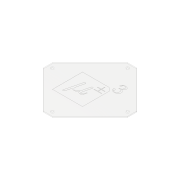
# Autodesk Inventor part: separatingPanels
Saved by Autodesk Inventor 2016 SP2 (Build 200236200, 236)
## iProperties
Created: 2016-07-21
Part Number: separatingPanels
Material: Polycarbonate, Clear
Document SubType Name: Modeling
Designer: Jonathan
Density: 1.2 g/cm^3
Appearance: Polycarbonate - Clear
Author: Jonathan
Autodesk Inventor part; units mm, degrees
(part 1 of 2)
ref_plane "YZ Plane" through (0, 0, 0) normal (1, 0, 0) x (0, 1, 0)
ref_plane "XZ Plane" through (0, 0, 0) normal (0, 1, 0) x (-1, 0, 0)
ref_plane "XY Plane" through (0, 0, 0) normal (0, 0, 1) x (1, 0, 0)
sketch "logo" plane through (0, 0, 0) normal (0, 0, 1) x (1, 0, 0)
  line L0 (123.8453, -88.283) -> (75.9446, -136.1837)
  line L1 (75.9446, -136.1837) -> (28.0439, -88.283)
  line L2 (28.0439, -88.283) -> (70.5564, -45.7705)
  spline S0 degree 3 poles (70.5564, -45.7705) (74.7474, -45.7705) (77.1417, -45.7705) (81.3327, -45.7705) knots 3 3 3 3 4 4 4 4
  line L3 (70.5564, -45.7705) -> (74.7474, -45.7705) construction
  line L4 (74.7474, -45.7705) -> (77.1417, -45.7705) construction
  line L5 (77.1417, -45.7705) -> (81.3327, -45.7705) construction
  line L6 (81.3327, -45.7705) -> (123.8453, -88.283)
  line L7 (135.6748, -1.3088) -> (16.9721, -1.3088)
  line L8 (16.9721, -1.3088) -> (1.3229, -16.958)
  line L9 (1.3229, -16.958) -> (1.3229, -135.6572)
  line L10 (1.3229, -135.6572) -> (16.9721, -151.3099)
  line L11 (16.9721, -151.3099) -> (135.6748, -151.3099)
  line L12 (135.6748, -151.3099) -> (151.324, -135.6572)
  line L13 (151.324, -135.6572) -> (151.324, -16.958)
  line L14 (151.324, -16.958) -> (135.6748, -1.3088)
  spline S1 degree 3 poles (16.2172, -139.1638) (14.7002, -139.1638) (13.4691, -137.9326) (13.4691, -136.4121) (13.4691, -134.8952) (14.7002, -133.664) (16.2172, -133.664) (17.7377, -133.664) (18.9689, -134.8952) (18.9689, -136.4121) (18.9689, -137.9326) (17.7377, -139.1638) (16.2172, -139.1638) knots 0 0 0 0 1 1 1 2 2 2 3 3 3 4 4 4 4
  line L15 (16.2172, -139.1638) -> (14.7002, -139.1638) construction
  line L16 (14.7002, -139.1638) -> (13.4691, -137.9326) construction
  line L17 (13.4691, -137.9326) -> (13.4691, -136.4121) construction
  line L18 (13.4691, -136.4121) -> (13.4691, -134.8952) construction
  line L19 (13.4691, -134.8952) -> (14.7002, -133.664) construction
  line L20 (14.7002, -133.664) -> (16.2172, -133.664) construction
  line L21 (16.2172, -133.664) -> (17.7377, -133.664) construction
  line L22 (17.7377, -133.664) -> (18.9689, -134.8952) construction
  line L23 (18.9689, -134.8952) -> (18.9689, -136.4121) construction
  line L24 (18.9689, -136.4121) -> (18.9689, -137.9326) construction
  line L25 (18.9689, -137.9326) -> (17.7377, -139.1638) construction
  line L26 (17.7377, -139.1638) -> (16.2172, -139.1638) construction
  spline S2 degree 3 poles (16.2172, -18.9547) (14.7002, -18.9547) (13.4691, -17.7236) (13.4691, -16.2031) (13.4691, -14.6861) (14.7002, -13.4549) (16.2172, -13.4549) (17.7377, -13.4549) (18.9689, -14.6861) (18.9689, -16.2031) (18.9689, -17.7236) (17.7377, -18.9547) (16.2172, -18.9547) knots 0 0 0 0 1 1 1 2 2 2 3 3 3 4 4 4 4
  line L27 (16.2172, -18.9547) -> (14.7002, -18.9547) construction
  line L28 (14.7002, -18.9547) -> (13.4691, -17.7236) construction
  line L29 (13.4691, -17.7236) -> (13.4691, -16.2031) construction
  line L30 (13.4691, -16.2031) -> (13.4691, -14.6861) construction
  line L31 (13.4691, -14.6861) -> (14.7002, -13.4549) construction
  line L32 (14.7002, -13.4549) -> (16.2172, -13.4549) construction
  line L33 (16.2172, -13.4549) -> (17.7377, -13.4549) construction
  line L34 (17.7377, -13.4549) -> (18.9689, -14.6861) construction
  line L35 (18.9689, -14.6861) -> (18.9689, -16.2031) construction
  line L36 (18.9689, -16.2031) -> (18.9689, -17.7236) construction
  line L37 (18.9689, -17.7236) -> (17.7377, -18.9547) construction
  line L38 (17.7377, -18.9547) -> (16.2172, -18.9547) construction
  spline S3 degree 3 poles (136.4262, -139.1638) (134.9093, -139.1638) (133.6781, -137.9326) (133.6781, -136.4121) (133.6781, -134.8952) (134.9093, -133.664) (136.4262, -133.664) (137.9467, -133.664) (139.1779, -134.8952) (139.1779, -136.4121) (139.1779, -137.9326) (137.9467, -139.1638) (136.4262, -139.1638) knots 0 0 0 0 1 1 1 2 2 2 3 3 3 4 4 4 4
  line L39 (136.4262, -139.1638) -> (134.9093, -139.1638) construction
  line L40 (134.9093, -139.1638) -> (133.6781, -137.9326) construction
  line L41 (133.6781, -137.9326) -> (133.6781, -136.4121) construction
  line L42 (133.6781, -136.4121) -> (133.6781, -134.8952) construction
  line L43 (133.6781, -134.8952) -> (134.9093, -133.664) construction
  line L44 (134.9093, -133.664) -> (136.4262, -133.664) construction
  line L45 (136.4262, -133.664) -> (137.9467, -133.664) construction
  line L46 (137.9467, -133.664) -> (139.1779, -134.8952) construction
  line L47 (139.1779, -134.8952) -> (139.1779, -136.4121) construction
  line L48 (139.1779, -136.4121) -> (139.1779, -137.9326) construction
  line L49 (139.1779, -137.9326) -> (137.9467, -139.1638) construction
  line L50 (137.9467, -139.1638) -> (136.4262, -139.1638) construction
  spline S4 degree 3 poles (136.4262, -18.9547) (134.9093, -18.9547) (133.6781, -17.7236) (133.6781, -16.2031) (133.6781, -14.6861) (134.9093, -13.4549) (136.4262, -13.4549) (137.9467, -13.4549) (139.1779, -14.6861) (139.1779, -16.2031) (139.1779, -17.7236) (137.9467, -18.9547) (136.4262, -18.9547) knots 0 0 0 0 1 1 1 2 2 2 3 3 3 4 4 4 4
  line L51 (136.4262, -18.9547) -> (134.9093, -18.9547) construction
  line L52 (134.9093, -18.9547) -> (133.6781, -17.7236) construction
  line L53 (133.6781, -17.7236) -> (133.6781, -16.2031) construction
  line L54 (133.6781, -16.2031) -> (133.6781, -14.6861) construction
  line L55 (133.6781, -14.6861) -> (134.9093, -13.4549) construction
  line L56 (134.9093, -13.4549) -> (136.4262, -13.4549) construction
  line L57 (136.4262, -13.4549) -> (137.9467, -13.4549) construction
  line L58 (137.9467, -13.4549) -> (139.1779, -14.6861) construction
  line L59 (139.1779, -14.6861) -> (139.1779, -16.2031) construction
  line L60 (139.1779, -16.2031) -> (139.1779, -17.7236) construction
  line L61 (139.1779, -17.7236) -> (137.9467, -18.9547) construction
  line L62 (137.9467, -18.9547) -> (136.4262, -18.9547) construction
  spline S5 degree 3 poles (62.3098, -86.8642) (61.6869, -85.6876) (60.3719, -83.542) (60.1643, -83.3344) knots 0 0 0 0 1 1 1 1
  line L63 (62.3098, -86.8642) -> (61.6869, -85.6876) construction
  line L64 (61.6869, -85.6876) -> (60.3719, -83.542) construction
  line L65 (60.3719, -83.542) -> (60.1643, -83.3344) construction
  spline S6 degree 3 poles (60.1643, -83.3344) (59.4029, -82.573) (58.434, -82.7115) (57.6726, -83.4728) knots 1 1 1 1 2 2 2 2
  line L66 (60.1643, -83.3344) -> (59.4029, -82.573) construction
  line L67 (59.4029, -82.573) -> (58.434, -82.7115) construction
  line L68 (58.434, -82.7115) -> (57.6726, -83.4728) construction
  spline S7 degree 3 poles (57.6726, -83.4728) (57.6034, -83.542) (56.4268, -84.857) (57.5342, -86.795) knots 2 2 2 2 3 3 3 3
  line L69 (57.6726, -83.4728) -> (57.6034, -83.542) construction
  line L70 (57.6034, -83.542) -> (56.4268, -84.857) construction
  line L71 (56.4268, -84.857) -> (57.5342, -86.795) construction
  line L72 (57.5342, -86.795) -> (76.7059, -118.7017)
  spline S8 degree 3 poles (76.7059, -118.7017) (77.1212, -119.3938) (77.1904, -119.463) (77.3288, -119.6015) knots 4 4 4 4 5 5 5 5
  line L73 (76.7059, -118.7017) -> (77.1212, -119.3938) construction
  line L74 (77.1212, -119.3938) -> (77.1904, -119.463) construction
  line L75 (77.1904, -119.463) -> (77.3288, -119.6015) construction
  spline S9 degree 3 poles (77.3288, -119.6015) (77.9517, -120.2244) (78.9899, -120.2936) (79.7513, -119.5322) (80.651, -118.6325) (80.3742, -117.2482) (80.3049, -117.0406) knots 5 5 5 5 6 6 6 7 7 7 7
  line L76 (77.3288, -119.6015) -> (77.9517, -120.2244) construction
  line L77 (77.9517, -120.2244) -> (78.9899, -120.2936) construction
  line L78 (78.9899, -120.2936) -> (79.7513, -119.5322) construction
  line L79 (79.7513, -119.5322) -> (80.651, -118.6325) construction
  line L80 (80.651, -118.6325) -> (80.3742, -117.2482) construction
  line L81 (80.3742, -117.2482) -> (80.3049, -117.0406) construction
  spline S10 degree 3 poles (80.3049, -117.0406) (80.1665, -116.4869) (78.367, -113.58) (73.2453, -105.1361) knots 7 7 7 7 8 8 8 8
  line L82 (80.3049, -117.0406) -> (80.1665, -116.4869) construction
  line L83 (80.1665, -116.4869) -> (78.367, -113.58) construction
  line L84 (78.367, -113.58) -> (73.2453, -105.1361) construction
  spline S11 degree 3 poles (73.2453, -105.1361) (75.8754, -104.8593) (78.0902, -103.0598) (78.9207, -102.2292) (82.0352, -99.1147) (81.7584, -95.3773) (81.5508, -93.0933) knots 8 8 8 8 9 9 9 10 10 10 10
  line L85 (73.2453, -105.1361) -> (75.8754, -104.8593) construction
  line L86 (75.8754, -104.8593) -> (78.0902, -103.0598) construction
  line L87 (78.0902, -103.0598) -> (78.9207, -102.2292) construction
  line L88 (78.9207, -102.2292) -> (82.0352, -99.1147) construction
  line L89 (82.0352, -99.1147) -> (81.7584, -95.3773) construction
  line L90 (81.7584, -95.3773) -> (81.5508, -93.0933) construction
  spline S12 degree 3 poles (81.5508, -93.0933) (83.9732, -94.6851) (86.8801, -94.2699) (88.818, -92.3319) (90.3407, -90.8093) (90.3407, -88.7329) (89.6486, -86.6565) knots 10 10 10 10 11 11 11 12 12 12 12
  line L91 (81.5508, -93.0933) -> (83.9732, -94.6851) construction
  line L92 (83.9732, -94.6851) -> (86.8801, -94.2699) construction
  line L93 (86.8801, -94.2699) -> (88.818, -92.3319) construction
  line L94 (88.818, -92.3319) -> (90.3407, -90.8093) construction
  line L95 (90.3407, -90.8093) -> (90.3407, -88.7329) construction
  line L96 (90.3407, -88.7329) -> (89.6486, -86.6565) construction
  spline S13 degree 3 poles (89.6486, -86.6565) (88.818, -84.3033) (86.6725, -81.0504) (86.6032, -80.9812) knots 12 12 12 12 13 13 13 13
  line L97 (89.6486, -86.6565) -> (88.818, -84.3033) construction
  line L98 (88.818, -84.3033) -> (86.6725, -81.0504) construction
  line L99 (86.6725, -81.0504) -> (86.6032, -80.9812) construction
  spline S14 degree 3 poles (86.6032, -80.9812) (86.1188, -80.4967) (85.7035, -80.9119) (85.5651, -81.0504) (85.1498, -81.4656) (85.2882, -81.7425) (85.7727, -82.5038) knots 13 13 13 13 14 14 14 15 15 15 15
  line L100 (86.6032, -80.9812) -> (86.1188, -80.4967) construction
  line L101 (86.1188, -80.4967) -> (85.7035, -80.9119) construction
  line L102 (85.7035, -80.9119) -> (85.5651, -81.0504) construction
  line L103 (85.5651, -81.0504) -> (85.1498, -81.4656) construction
  line L104 (85.1498, -81.4656) -> (85.2882, -81.7425) construction
  line L105 (85.2882, -81.7425) -> (85.7727, -82.5038) construction
  spline S15 degree 3 poles (85.7727, -82.5038) (87.9183, -86.0336) (89.7178, -89.4942) (87.9183, -91.2937) (86.7417, -92.4703) (85.4266, -91.4322) (84.5961, -90.6016) (83.6271, -89.6327) (82.0352, -87.0718) (80.7894, -85.1339) knots 15 15 15 15 16 16 16 17 17 17 18 18 18 18
  line L106 (85.7727, -82.5038) -> (87.9183, -86.0336) construction
  line L107 (87.9183, -86.0336) -> (89.7178, -89.4942) construction
  line L108 (89.7178, -89.4942) -> (87.9183, -91.2937) construction
  line L109 (87.9183, -91.2937) -> (86.7417, -92.4703) construction
  line L110 (86.7417, -92.4703) -> (85.4266, -91.4322) construction
  line L111 (85.4266, -91.4322) -> (84.5961, -90.6016) construction
  line L112 (84.5961, -90.6016) -> (83.6271, -89.6327) construction
  line L113 (83.6271, -89.6327) -> (82.0352, -87.0718) construction
  line L114 (82.0352, -87.0718) -> (80.7894, -85.1339) construction
  line L115 (80.7894, -85.1339) -> (77.2596, -79.1124)
  spline S16 degree 3 poles (77.2596, -79.1124) (76.7751, -78.3511) (75.5985, -76.2055) (75.0448, -75.375) (74.2143, -74.1292) (73.0377, -71.9836) (72.7608, -71.7068) knots 19 19 19 19 20 20 20 21 21 21 21
  line L116 (77.2596, -79.1124) -> (76.7751, -78.3511) construction
  line L117 (76.7751, -78.3511) -> (75.5985, -76.2055) construction
  line L118 (75.5985, -76.2055) -> (75.0448, -75.375) construction
  line L119 (75.0448, -75.375) -> (74.2143, -74.1292) construction
  line L120 (74.2143, -74.1292) -> (73.0377, -71.9836) construction
  line L121 (73.0377, -71.9836) -> (72.7608, -71.7068) construction
  spline S17 degree 3 poles (72.7608, -71.7068) (71.9995, -70.9454) (70.9613, -71.1531) (70.2692, -71.8452) (70.0616, -72.0528) (68.9542, -73.2986) (70.0616, -75.0981) knots 21 21 21 21 22 22 22 23 23 23 23
  line L122 (72.7608, -71.7068) -> (71.9995, -70.9454) construction
  line L123 (71.9995, -70.9454) -> (70.9613, -71.1531) construction
  line L124 (70.9613, -71.1531) -> (70.2692, -71.8452) construction
  line L125 (70.2692, -71.8452) -> (70.0616, -72.0528) construction
  line L126 (70.0616, -72.0528) -> (68.9542, -73.2986) construction
  line L127 (68.9542, -73.2986) -> (70.0616, -75.0981) construction
  line L128 (70.0616, -75.0981) -> (76.2907, -85.4799)
  spline S18 degree 3 poles (76.2907, -85.4799) (78.021, -88.1792) (79.336, -90.4632) (79.682, -91.0861) knots 24 24 24 24 25 25 25 25
  line L129 (76.2907, -85.4799) -> (78.021, -88.1792) construction
  line L130 (78.021, -88.1792) -> (79.336, -90.4632) construction
  line L131 (79.336, -90.4632) -> (79.682, -91.0861) construction
  spline S19 degree 3 poles (79.682, -91.0861) (79.8205, -91.363) (81.7584, -97.4536) (78.1594, -101.0526) (75.9446, -103.2674) (73.453, -102.8521) (71.0305, -100.4297) (69.7847, -99.1839) (68.8158, -97.6612) (67.916, -96.0694) knots 25 25 25 25 26 26 26 27 27 27 28 28 28 28
  line L132 (79.682, -91.0861) -> (79.8205, -91.363) construction
  line L133 (79.8205, -91.363) -> (81.7584, -97.4536) construction
  line L134 (81.7584, -97.4536) -> (78.1594, -101.0526) construction
  line L135 (78.1594, -101.0526) -> (75.9446, -103.2674) construction
  line L136 (75.9446, -103.2674) -> (73.453, -102.8521) construction
  line L137 (73.453, -102.8521) -> (71.0305, -100.4297) construction
  line L138 (71.0305, -100.4297) -> (69.7847, -99.1839) construction
  line L139 (69.7847, -99.1839) -> (68.8158, -97.6612) construction
  line L140 (68.8158, -97.6612) -> (67.916, -96.0694) construction
  line L141 (67.916, -96.0694) -> (62.3098, -86.8642)
  line L142 (76.7453, -58.3124) -> (81.6949, -53.3628)
  spline S20 degree 3 poles (81.6949, -53.3628) (81.9496, -53.1081) (82.3136, -52.7441) (81.9132, -52.3438) knots 1 1 1 1 2 2 2 2
  line L143 (81.6949, -53.3628) -> (81.9496, -53.1081) construction
  line L144 (81.9496, -53.1081) -> (82.3136, -52.7441) construction
  line L145 (82.3136, -52.7441) -> (81.9132, -52.3438) construction
  spline S21 degree 3 poles (81.9132, -52.3438) (81.5129, -51.9435) (81.149, -52.3074) (80.8942, -52.5622) knots 2 2 2 2 3 3 3 3
  line L146 (81.9132, -52.3438) -> (81.5129, -51.9435) construction
  line L147 (81.5129, -51.9435) -> (81.149, -52.3074) construction
  line L148 (81.149, -52.3074) -> (80.8942, -52.5622) construction
  line L149 (80.8942, -52.5622) -> (75.9446, -57.5118)
  line L150 (75.9446, -57.5118) -> (71.0678, -52.635)
  spline S22 degree 3 poles (71.0678, -52.635) (70.7766, -52.3438) (70.3763, -51.9435) (69.976, -52.3438) (69.5756, -52.7441) (69.9396, -53.1081) (70.1943, -53.3628) knots 5 5 5 5 6 6 6 7 7 7 7
  line L151 (71.0678, -52.635) -> (70.7766, -52.3438) construction
  line L152 (70.7766, -52.3438) -> (70.3763, -51.9435) construction
  line L153 (70.3763, -51.9435) -> (69.976, -52.3438) construction
  line L154 (69.976, -52.3438) -> (69.5756, -52.7441) construction
  line L155 (69.5756, -52.7441) -> (69.9396, -53.1081) construction
  line L156 (69.9396, -53.1081) -> (70.1943, -53.3628) construction
  line L157 (70.1943, -53.3628) -> (75.1439, -58.3124)
  line L158 (75.1439, -58.3124) -> (70.1943, -63.262)
  spline S23 degree 3 poles (70.1943, -63.262) (69.9396, -63.5168) (69.5392, -63.9171) (69.9396, -64.3175) knots 9 9 9 9 10 10 10 10
  line L159 (70.1943, -63.262) -> (69.9396, -63.5168) construction
  line L160 (69.9396, -63.5168) -> (69.5392, -63.9171) construction
  line L161 (69.5392, -63.9171) -> (69.9396, -64.3175) construction
  spline S24 degree 3 poles (69.9396, -64.3175) (70.3399, -64.7178) (70.7402, -64.3175) (70.995, -64.0627) knots 10 10 10 10 11 11 11 11
  line L162 (69.9396, -64.3175) -> (70.3399, -64.7178) construction
  line L163 (70.3399, -64.7178) -> (70.7402, -64.3175) construction
  line L164 (70.7402, -64.3175) -> (70.995, -64.0627) construction
  line L165 (70.995, -64.0627) -> (75.9446, -59.1131)
  line L166 (75.9446, -59.1131) -> (80.7486, -63.9171)
  line L167 (80.7486, -63.9171) -> (75.799, -68.8667)
  spline S25 degree 3 poles (75.799, -68.8667) (75.5443, -69.1215) (75.1439, -69.5218) (75.5443, -69.9222) knots 14 14 14 14 15 15 15 15
  line L168 (75.799, -68.8667) -> (75.5443, -69.1215) construction
  line L169 (75.5443, -69.1215) -> (75.1439, -69.5218) construction
  line L170 (75.1439, -69.5218) -> (75.5443, -69.9222) construction
  spline S26 degree 3 poles (75.5443, -69.9222) (75.9446, -70.3225) (76.3449, -69.9222) (76.5997, -69.6674) knots 15 15 15 15 16 16 16 16
  line L171 (75.5443, -69.9222) -> (75.9446, -70.3225) construction
  line L172 (75.9446, -70.3225) -> (76.3449, -69.9222) construction
  line L173 (76.3449, -69.9222) -> (76.5997, -69.6674) construction
  line L174 (76.5997, -69.6674) -> (87.2996, -58.9675)
  spline S27 degree 3 poles (87.2996, -58.9675) (87.5543, -58.7128) (87.9183, -58.3488) (87.5179, -57.9485) knots 17 17 17 17 18 18 18 18
  line L175 (87.2996, -58.9675) -> (87.5543, -58.7128) construction
  line L176 (87.5543, -58.7128) -> (87.9183, -58.3488) construction
  line L177 (87.9183, -58.3488) -> (87.5179, -57.9485) construction
  spline S28 degree 3 poles (87.5179, -57.9485) (87.1176, -57.5482) (86.7537, -57.9121) (86.4989, -58.1669) knots 18 18 18 18 19 19 19 19
  line L178 (87.5179, -57.9485) -> (87.1176, -57.5482) construction
  line L179 (87.1176, -57.5482) -> (86.7537, -57.9121) construction
  line L180 (86.7537, -57.9121) -> (86.4989, -58.1669) construction
  line L181 (86.4989, -58.1669) -> (81.5493, -63.1165)
  line L182 (81.5493, -63.1165) -> (76.7453, -58.3124)
  spline S29 degree 3 poles (75.3605, -28.3562) (77.4048, -26.312) (80.2668, -26.2535) (83.0704, -29.0571) (86.2828, -32.2696) (85.3483, -35.19) (83.8881, -36.6502) (82.8368, -37.7015) (80.2084, -39.7458) (77.58, -39.2202) knots 0 0 0 0 1 1 1 2 2 2 3 3 3 3
  line L183 (75.3605, -28.3562) -> (77.4048, -26.312) construction
  line L184 (77.4048, -26.312) -> (80.2668, -26.2535) construction
  line L185 (80.2668, -26.2535) -> (83.0704, -29.0571) construction
  line L186 (83.0704, -29.0571) -> (86.2828, -32.2696) construction
  line L187 (86.2828, -32.2696) -> (85.3483, -35.19) construction
  line L188 (85.3483, -35.19) -> (83.8881, -36.6502) construction
  line L189 (83.8881, -36.6502) -> (82.8368, -37.7015) construction
  line L190 (82.8368, -37.7015) -> (80.2084, -39.7458) construction
  line L191 (80.2084, -39.7458) -> (77.58, -39.2202) construction
  spline S30 degree 3 poles (77.58, -39.2202) (78.8066, -37.9936) (78.2225, -36.8254) (77.6384, -36.2413) (76.8207, -35.4236) (75.5941, -35.482) (74.7764, -36.2998) (74.0755, -37.0007) (73.7835, -38.2272) (74.8348, -39.2786) (77.288, -41.7317) (81.5518, -40.622) (84.7058, -37.4679) (88.3271, -33.8466) (88.3855, -28.8819) (85.8156, -26.312) (83.7713, -24.2677) (80.0916, -23.8588) (76.6455, -26.1367) knots 3 3 3 3 4 4 4 5 5 5 6 6 6 7 7 7 8 8 8 9 9 9 9
  line L192 (77.58, -39.2202) -> (78.8066, -37.9936) construction
  line L193 (78.8066, -37.9936) -> (78.2225, -36.8254) construction
  line L194 (78.2225, -36.8254) -> (77.6384, -36.2413) construction
  line L195 (77.6384, -36.2413) -> (76.8207, -35.4236) construction
  line L196 (76.8207, -35.4236) -> (75.5941, -35.482) construction
  line L197 (75.5941, -35.482) -> (74.7764, -36.2998) construction
  line L198 (74.7764, -36.2998) -> (74.0755, -37.0007) construction
  line L199 (74.0755, -37.0007) -> (73.7835, -38.2272) construction
  line L200 (73.7835, -38.2272) -> (74.8348, -39.2786) construction
  line L201 (74.8348, -39.2786) -> (77.288, -41.7317) construction
  line L202 (77.288, -41.7317) -> (81.5518, -40.622) construction
  line L203 (81.5518, -40.622) -> (84.7058, -37.4679) construction
  line L204 (84.7058, -37.4679) -> (88.3271, -33.8466) construction
  line L205 (88.3271, -33.8466) -> (88.3855, -28.8819) construction
  line L206 (88.3855, -28.8819) -> (85.8156, -26.312) construction
  line L207 (85.8156, -26.312) -> (83.7713, -24.2677) construction
  line L208 (83.7713, -24.2677) -> (80.0916, -23.8588) construction
  line L209 (80.0916, -23.8588) -> (76.6455, -26.1367) construction
  spline S31 degree 3 poles (76.6455, -26.1367) (78.3393, -22.457) (77.4048, -19.5366) (75.7694, -17.9012) (73.7251, -15.8569) (69.8701, -16.6746) (66.9497, -19.595) (64.0877, -22.457) (63.27, -26.0783) (65.3727, -28.181) (66.2488, -29.0571) (67.3002, -28.9403) (68.0595, -28.181) (68.8772, -27.3633) (68.8188, -26.2535) (68.1179, -25.5526) (67.3586, -24.7933) (66.2488, -24.7349) (65.3727, -25.4942) knots 9 9 9 9 10 10 10 11 11 11 12 12 12 13 13 13 14 14 14 15 15 15 15
  line L210 (76.6455, -26.1367) -> (78.3393, -22.457) construction
  line L211 (78.3393, -22.457) -> (77.4048, -19.5366) construction
  line L212 (77.4048, -19.5366) -> (75.7694, -17.9012) construction
  line L213 (75.7694, -17.9012) -> (73.7251, -15.8569) construction
  line L214 (73.7251, -15.8569) -> (69.8701, -16.6746) construction
  line L215 (69.8701, -16.6746) -> (66.9497, -19.595) construction
  line L216 (66.9497, -19.595) -> (64.0877, -22.457) construction
  line L217 (64.0877, -22.457) -> (63.27, -26.0783) construction
  line L218 (63.27, -26.0783) -> (65.3727, -28.181) construction
  line L219 (65.3727, -28.181) -> (66.2488, -29.0571) construction
  line L220 (66.2488, -29.0571) -> (67.3002, -28.9403) construction
  line L221 (67.3002, -28.9403) -> (68.0595, -28.181) construction
  line L222 (68.0595, -28.181) -> (68.8772, -27.3633) construction
  line L223 (68.8772, -27.3633) -> (68.8188, -26.2535) construction
  line L224 (68.8188, -26.2535) -> (68.1179, -25.5526) construction
  line L225 (68.1179, -25.5526) -> (67.3586, -24.7933) construction
  line L226 (67.3586, -24.7933) -> (66.2488, -24.7349) construction
  line L227 (66.2488, -24.7349) -> (65.3727, -25.4942) construction
  spline S32 degree 3 poles (65.3727, -25.4942) (65.1975, -23.45) (66.6577, -21.4057) (67.6506, -20.4127) (68.8188, -19.2446) (71.0383, -18.1932) (73.2578, -20.4127) (74.3676, -21.5225) (75.2437, -23.0995) (75.3021, -24.5597) knots 15 15 15 15 16 16 16 17 17 17 18 18 18 18
  line L228 (65.3727, -25.4942) -> (65.1975, -23.45) construction
  line L229 (65.1975, -23.45) -> (66.6577, -21.4057) construction
  line L230 (66.6577, -21.4057) -> (67.6506, -20.4127) construction
  line L231 (67.6506, -20.4127) -> (68.8188, -19.2446) construction
  line L232 (68.8188, -19.2446) -> (71.0383, -18.1932) construction
  line L233 (71.0383, -18.1932) -> (73.2578, -20.4127) construction
  line L234 (73.2578, -20.4127) -> (74.3676, -21.5225) construction
  line L235 (74.3676, -21.5225) -> (75.2437, -23.0995) construction
  line L236 (75.2437, -23.0995) -> (75.3021, -24.5597) construction
  spline S33 degree 3 poles (75.3021, -24.5597) (75.4773, -26.3704) (74.7764, -27.1881) (73.6083, -28.5899) (73.0242, -29.2908) (72.9658, -29.3492) (72.849, -29.466) (72.7906, -29.5244) (72.6153, -29.8164) (72.9074, -30.1085) knots 18 18 18 18 19 19 19 20 20 20 21 21 21 21
  line L237 (75.3021, -24.5597) -> (75.4773, -26.3704) construction
  line L238 (75.4773, -26.3704) -> (74.7764, -27.1881) construction
  line L239 (74.7764, -27.1881) -> (73.6083, -28.5899) construction
  line L240 (73.6083, -28.5899) -> (73.0242, -29.2908) construction
  line L241 (73.0242, -29.2908) -> (72.9658, -29.3492) construction
  line L242 (72.9658, -29.3492) -> (72.849, -29.466) construction
  line L243 (72.849, -29.466) -> (72.7906, -29.5244) construction
  line L244 (72.7906, -29.5244) -> (72.6153, -29.8164) construction
  line L245 (72.6153, -29.8164) -> (72.9074, -30.1085) construction
  spline S34 degree 3 poles (72.9074, -30.1085) (73.2578, -30.4589) (73.4914, -30.2253) (73.9587, -29.758) knots 21 21 21 21 22 22 22 22
  line L246 (72.9074, -30.1085) -> (73.2578, -30.4589) construction
  line L247 (73.2578, -30.4589) -> (73.4914, -30.2253) construction
  line L248 (73.4914, -30.2253) -> (73.9587, -29.758) construction
  line L249 (73.9587, -29.758) -> (75.3605, -28.3562)
  point P0 (76.1833, -66.2121)
sketch "mu" plane through (0, 0, 0) normal (0, 0, 1) x (1, 0, 0)
  spline S0 degree 3 poles (-17.3729, 2.4446) (-16.9814, 3.7171) (-16.3941, 6.1641) (-16.3941, 6.4577) knots 0 0 0 0 1 1 1 1
  line L0 (-17.3729, 2.4446) -> (-16.9814, 3.7171) construction
  line L1 (-16.9814, 3.7171) -> (-16.3941, 6.1641) construction
  line L2 (-16.3941, 6.1641) -> (-16.3941, 6.4577) construction
  spline S1 degree 3 poles (-16.3941, 6.4577) (-16.3941, 7.5344) (-17.1772, 8.1217) (-18.2539, 8.1217) knots 1 1 1 1 2 2 2 2
  line L3 (-16.3941, 6.4577) -> (-16.3941, 7.5344) construction
  line L4 (-16.3941, 7.5344) -> (-17.1772, 8.1217) construction
  line L5 (-17.1772, 8.1217) -> (-18.2539, 8.1217) construction
  spline S2 degree 3 poles (-18.2539, 8.1217) (-18.3517, 8.1217) (-20.1136, 8.0238) (-20.7009, 5.8705) knots 2 2 2 2 3 3 3 3
  line L6 (-18.2539, 8.1217) -> (-18.3517, 8.1217) construction
  line L7 (-18.3517, 8.1217) -> (-20.1136, 8.0238) construction
  line L8 (-20.1136, 8.0238) -> (-20.7009, 5.8705) construction
  line L9 (-20.7009, 5.8705) -> (-29.7059, -30.2475)
  spline S3 degree 3 poles (-29.7059, -30.2475) (-29.9017, -31.0305) (-29.9017, -31.1284) (-29.9017, -31.3241) knots 4 4 4 4 5 5 5 5
  line L10 (-29.7059, -30.2475) -> (-29.9017, -31.0305) construction
  line L11 (-29.9017, -31.0305) -> (-29.9017, -31.1284) construction
  line L12 (-29.9017, -31.1284) -> (-29.9017, -31.3241) construction
  spline S4 degree 3 poles (-29.9017, -31.3241) (-29.9017, -32.2051) (-29.2165, -32.9881) (-28.1398, -32.9881) (-26.8674, -32.9881) (-26.0843, -31.8136) (-25.9864, -31.6178) knots 5 5 5 5 6 6 6 7 7 7 7
  line L13 (-29.9017, -31.3241) -> (-29.9017, -32.2051) construction
  line L14 (-29.9017, -32.2051) -> (-29.2165, -32.9881) construction
  line L15 (-29.2165, -32.9881) -> (-28.1398, -32.9881) construction
  line L16 (-28.1398, -32.9881) -> (-26.8674, -32.9881) construction
  line L17 (-26.8674, -32.9881) -> (-26.0843, -31.8136) construction
  line L18 (-26.0843, -31.8136) -> (-25.9864, -31.6178) construction
  spline S5 degree 3 poles (-25.9864, -31.6178) (-25.6928, -31.1284) (-24.9098, -27.8004) (-22.5606, -18.2082) knots 7 7 7 7 8 8 8 8
  line L19 (-25.9864, -31.6178) -> (-25.6928, -31.1284) construction
  line L20 (-25.6928, -31.1284) -> (-24.9098, -27.8004) construction
  line L21 (-24.9098, -27.8004) -> (-22.5606, -18.2082) construction
  spline S6 degree 3 poles (-22.5606, -18.2082) (-20.5051, -19.8721) (-17.6666, -20.1658) (-16.492, -20.1658) (-12.0874, -20.1658) (-9.6404, -17.3272) (-8.1722, -15.5654) knots 8 8 8 8 9 9 9 10 10 10 10
  line L22 (-22.5606, -18.2082) -> (-20.5051, -19.8721) construction
  line L23 (-20.5051, -19.8721) -> (-17.6666, -20.1658) construction
  line L24 (-17.6666, -20.1658) -> (-16.492, -20.1658) construction
  line L25 (-16.492, -20.1658) -> (-12.0874, -20.1658) construction
  line L26 (-12.0874, -20.1658) -> (-9.6404, -17.3272) construction
  line L27 (-9.6404, -17.3272) -> (-8.1722, -15.5654) construction
  spline S7 degree 3 poles (-8.1722, -15.5654) (-7.5849, -18.4039) (-5.2358, -20.1658) (-2.4951, -20.1658) (-0.3417, -20.1658) (1.1265, -18.6976) (2.1053, -16.74) knots 10 10 10 10 11 11 11 12 12 12 12
  line L28 (-8.1722, -15.5654) -> (-7.5849, -18.4039) construction
  line L29 (-7.5849, -18.4039) -> (-5.2358, -20.1658) construction
  line L30 (-5.2358, -20.1658) -> (-2.4951, -20.1658) construction
  line L31 (-2.4951, -20.1658) -> (-0.3417, -20.1658) construction
  line L32 (-0.3417, -20.1658) -> (1.1265, -18.6976) construction
  line L33 (1.1265, -18.6976) -> (2.1053, -16.74) construction
  spline S8 degree 3 poles (2.1053, -16.74) (3.182, -14.4887) (3.965, -10.6714) (3.965, -10.5735) knots 12 12 12 12 13 13 13 13
  line L34 (2.1053, -16.74) -> (3.182, -14.4887) construction
  line L35 (3.182, -14.4887) -> (3.965, -10.6714) construction
  line L36 (3.965, -10.6714) -> (3.965, -10.5735) construction
  spline S9 degree 3 poles (3.965, -10.5735) (3.965, -9.8883) (3.3777, -9.8883) (3.182, -9.8883) (2.5947, -9.8883) (2.4968, -10.182) (2.301, -11.0629) knots 13 13 13 13 14 14 14 15 15 15 15
  line L37 (3.965, -10.5735) -> (3.965, -9.8883) construction
  line L38 (3.965, -9.8883) -> (3.3777, -9.8883) construction
  line L39 (3.3777, -9.8883) -> (3.182, -9.8883) construction
  line L40 (3.182, -9.8883) -> (2.5947, -9.8883) construction
  line L41 (2.5947, -9.8883) -> (2.4968, -10.182) construction
  line L42 (2.4968, -10.182) -> (2.301, -11.0629) construction
  spline S10 degree 3 poles (2.301, -11.0629) (1.3222, -15.076) (0.1477, -18.7955) (-2.3972, -18.7955) (-4.0612, -18.7955) (-4.257, -17.1315) (-4.257, -15.9569) (-4.257, -14.5866) (-3.5718, -11.6502) (-3.0824, -9.3989) knots 15 15 15 15 16 16 16 17 17 17 18 18 18 18
  line L43 (2.301, -11.0629) -> (1.3222, -15.076) construction
  line L44 (1.3222, -15.076) -> (0.1477, -18.7955) construction
  line L45 (0.1477, -18.7955) -> (-2.3972, -18.7955) construction
  line L46 (-2.3972, -18.7955) -> (-4.0612, -18.7955) construction
  line L47 (-4.0612, -18.7955) -> (-4.257, -17.1315) construction
  line L48 (-4.257, -17.1315) -> (-4.257, -15.9569) construction
  line L49 (-4.257, -15.9569) -> (-4.257, -14.5866) construction
  line L50 (-4.257, -14.5866) -> (-3.5718, -11.6502) construction
  line L51 (-3.5718, -11.6502) -> (-3.0824, -9.3989) construction
  line L52 (-3.0824, -9.3989) -> (-1.3205, -2.6452)
  spline S11 degree 3 poles (-1.3205, -2.6452) (-1.1248, -1.7642) (-0.4396, 0.5849) (-0.2438, 1.5637) (0.0498, 3.0319) (0.735, 5.381) (0.735, 5.7726) knots 19 19 19 19 20 20 20 21 21 21 21
  line L53 (-1.3205, -2.6452) -> (-1.1248, -1.7642) construction
  line L54 (-1.1248, -1.7642) -> (-0.4396, 0.5849) construction
  line L55 (-0.4396, 0.5849) -> (-0.2438, 1.5637) construction
  line L56 (-0.2438, 1.5637) -> (0.0498, 3.0319) construction
  line L57 (0.0498, 3.0319) -> (0.735, 5.381) construction
  line L58 (0.735, 5.381) -> (0.735, 5.7726) construction
  spline S12 degree 3 poles (0.735, 5.7726) (0.735, 6.8492) (-0.146, 7.4365) (-1.1248, 7.4365) (-1.4184, 7.4365) (-3.0824, 7.3386) (-3.5718, 5.2832) knots 21 21 21 21 22 22 22 23 23 23 23
  line L59 (0.735, 5.7726) -> (0.735, 6.8492) construction
  line L60 (0.735, 6.8492) -> (-0.146, 7.4365) construction
  line L61 (-0.146, 7.4365) -> (-1.1248, 7.4365) construction
  line L62 (-1.1248, 7.4365) -> (-1.4184, 7.4365) construction
  line L63 (-1.4184, 7.4365) -> (-3.0824, 7.3386) construction
  line L64 (-3.0824, 7.3386) -> (-3.5718, 5.2832) construction
  line L65 (-3.5718, 5.2832) -> (-6.5082, -6.4625)
  spline S13 degree 3 poles (-6.5082, -6.4625) (-7.1934, -9.5947) (-7.8785, -12.1396) (-8.0743, -12.8247) knots 24 24 24 24 25 25 25 25
  line L66 (-6.5082, -6.4625) -> (-7.1934, -9.5947) construction
  line L67 (-7.1934, -9.5947) -> (-7.8785, -12.1396) construction
  line L68 (-7.8785, -12.1396) -> (-8.0743, -12.8247) construction
  spline S14 degree 3 poles (-8.0743, -12.8247) (-8.1722, -13.1184) (-11.1086, -18.7954) (-16.1984, -18.7954) (-19.3306, -18.7954) (-20.7988, -16.74) (-20.7988, -13.3141) (-20.7988, -11.5523) (-20.4072, -9.7904) (-19.9178, -8.0286) knots 25 25 25 25 26 26 26 27 27 27 28 28 28 28
  line L69 (-8.0743, -12.8247) -> (-8.1722, -13.1184) construction
  line L70 (-8.1722, -13.1184) -> (-11.1086, -18.7954) construction
  line L71 (-11.1086, -18.7954) -> (-16.1984, -18.7954) construction
  line L72 (-16.1984, -18.7954) -> (-19.3306, -18.7954) construction
  line L73 (-19.3306, -18.7954) -> (-20.7988, -16.74) construction
  line L74 (-20.7988, -16.74) -> (-20.7988, -13.3141) construction
  line L75 (-20.7988, -13.3141) -> (-20.7988, -11.5523) construction
  line L76 (-20.7988, -11.5523) -> (-20.4072, -9.7904) construction
  line L77 (-20.4072, -9.7904) -> (-19.9178, -8.0286) construction
  line L78 (-19.9178, -8.0286) -> (-17.3729, 2.4446)
  point P0 (-10.6472, -11.2008)
sketch "Sketch1" plane through (0, 0, 0) normal (0, 1, 0) x (-1, 0, 0)
  line L0 (95, -95) -> (-95, -95)
  line L1 (-95, -95) -> (-95, 95)
  line L2 (-95, 95) -> (95, 95)
  line L3 (95, 95) -> (95, -95)
  line L4 (95, -95) -> (-95, 95) construction
  line L5 (-95, -95) -> (95, 95) construction
  point P0 (0, 0)
  point P1 (0, 0)
  point P2 (0, 0)
  dimension "d25" = 190
  constraints: 12 end point, 3 midpoint, 2 parallel, 2 perpendicular, 1 coincident, 1 horizontal
  measures "d25" distance of L0.end L1.end
extrude "Extrusion1" add sketch "Sketch1" along normal blind 2.3813
sketch "Sketch2" plane through (0, 2.3813, 0) normal (0, 1, 0) x (1, 0, 0)
  line L0 (-95, -95) -> (95, -95) projected
  point P0 (0, 0)
  point P1 (0, -85)
  dimension "d26" = 10
  constraints: 1 vertical alignment
  measures "d26" distance from line of L0 point (0, -85)
hole "Hole1" at (0, 2.3813, 85) direction (0, -1, 0) diameter 5.5 end through all clearance for "Socket Head Cap Screw" size "M5" standard "Ansi Metric M Profile"
pattern_circular "Circular Pattern1" count 4 over 360 about axis through (0, -10, 0) along (0, 1, 0) of "Hole1"
sketch "Sketch3" plane through (0, 0, 0) normal (0, -1, 0) x (1, 0, 0)
  circle A0 centre (-85, 0) radius 2.75 projected
  circle A1 centre (0, -85) radius 2.75 projected
  circle A2 centre (85, 0) radius 2.75 projected
  circle A3 centre (0, 85) radius 2.75 projected
  line L0 (-95, -95) -> (95, -95) projected
  line L1 (95, -95) -> (95, 95) projected
  line L2 (95, 95) -> (-95, 95) projected
  line L3 (-95, 95) -> (-95, -95) projected
  line L4 (0, 106.066) -> (106.066, 0)
  line L5 (106.066, 0) -> (0, -106.066)
  line L6 (0, -106.066) -> (-106.066, 0)
  line L7 (-106.066, 0) -> (0, 106.066)
  line L8 (-106.066, 0) -> (106.066, 0) construction
  line L9 (0, -106.066) -> (0, 106.066) construction
  point P0 (0, 0)
  point P1 (0, 0)
  point P2 (0, 0)
  dimension "d27" = 150
  dimension "d28" = 150
  constraints: 12 end point, 2 midpoint, 2 parallel, 1 coincident, 1 horizontal, 1 perpendicular
  measures "d27" distance between parallel lines of L7 L5
  measures "d28" distance between parallel lines of L6 L4
extrude "Extrusion2" cut sketch "Sketch3" against normal through all contours L6 L3 L7 L2 L4 L1 L5 L0 | L0 L5 L6 | L6 L7 L3 | L1 L4 L5 | L7 L4 L2 keep common part